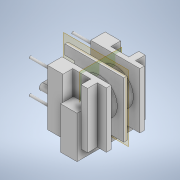
# Autodesk Inventor part: UU10.5Y
Saved by Autodesk Inventor 2020 (Build 240168000, 168)
## iProperties
Created: 2021-07-21
Part Number: UU10.5Y
Material: Типовые
Document SubType Name: Modeling
Designer: VB
Density: 1 g/cm^3
Appearance: По умолчанию
Author: VB
Autodesk Inventor part; units mm, degrees
ref_plane "YZ Plane" through (0, 0, 0) normal (1, 0, 0) x (0, 1, 0)
ref_plane "XZ Plane" through (0, 0, 0) normal (0, 1, 0) x (-1, 0, 0)
ref_plane "XY Plane" through (0, 0, 0) normal (0, 0, 1) x (1, 0, 0)
sketch "Эскиз1" plane through (0, 0, 0) normal (0, 1, 0) x (-1, 0, 0)
  line L0 (9, 8.8) -> (9, -8.8) construction
  line L1 (-9, -8.8) -> (-9, 8.8) construction
  line L2 (-9, 8.8) -> (9, -8.8) construction
  line L3 (9, 8.8) -> (-9, -8.8) construction
  line L4 (9, 0) -> (9, 0.5)
  line L5 (9, 0.5) -> (-9, 0.5)
  line L6 (9, 0) -> (9, -0.4719)
  line L7 (9, -0.4719) -> (-9, -0.4719)
  line L8 (-9, 0.5) -> (-9, -0.4719)
  line L9 (9, 0) -> (9, 4.3404) construction
  line L10 (9, 0) -> (9, -4.4046) construction
  line L11 (9, 4.3404) -> (-9, 4.3404)
  line L12 (-9, 4.3404) -> (-9, 8.8)
  line L13 (-9, 8.8) -> (9, 8.8)
  line L14 (9, 8.8) -> (9, 4.3404)
  line L15 (9, -4.4046) -> (-9, -4.4046)
  line L16 (-9, -4.4046) -> (-9, -8.8)
  line L17 (-9, -8.8) -> (9, -8.8)
  line L18 (9, -8.8) -> (9, -4.4046)
  point P0 (0, 0)
  dimension "d0" = 18
  dimension "d1" = 17.6
  dimension "d2" = 0.5
  constraints: 38 end point, 6 point on line, 5 parallel, 4 perpendicular, 3 midpoint, 2 horizontal, 1 collinear
  measures "d0" distance of L0.end L1.start
  measures "d1" distance of L0.start L0.end
  measures "d2" distance of L4.start L4.end
extrude "Выдавливание1" add sketch "Эскиз1" along normal blind 17
sketch "Эскиз6" plane through (9, 0, 4.3404) normal (0, 0, -1) x (-1, 0, 0)
  line L0 (9, 0) -> (9, 17) construction
  line L1 (18, 17) -> (0, 17) projected
  line L2 (9, 8.5) -> (7.5, 8.5) construction
  circle A0 centre (7.5, 8.5) radius 5.5
  dimension "d16" = 1.5
  dimension "d53" = 11
  constraints: 4 end point, 2 midpoint, 1 centre point, 1 coincident, 1 horizontal
  measures "d16" distance of L2.start L2.end
  measures "d53" diameter of A0
extrude "Выдавливание3" add sketch "Эскиз6" along normal up to surface (8.745 mm away)
sketch "Эскиз10" plane through (-9, 0, 4.3404) normal (-1, 0, 0) x (0, 0, 1)
  line L0 (4.4596, 6.45) -> (4.4596, 11.95) projected
  line L1 (4.4596, 9.2) -> (-13.9375, 9.2) construction
  line L2 (-14.0763, 11.7) -> (-14.0763, 6.7) projected
  line L3 (1, 9.2) -> (2.9596, 9.2) construction
  line L4 (1, 8.2) -> (2.9596, 8.2)
  line L5 (2.9596, 10.2) -> (1, 10.2)
  arc A0 (1, 10.2) -> (1, 8.2) centre (1, 9.2) ccw
  arc A1 (2.9596, 8.2) -> (2.9596, 10.2) centre (2.9596, 9.2) ccw
  line L6 (0, 0) -> (0, 17) projected
  line L7 (4.4596, 0) -> (4.4596, 17) projected
  line L8 (-9.745, 9.2) -> (-11.6404, 9.2) construction
  line L9 (-9.745, 10.2) -> (-11.6404, 10.2)
  line L10 (-11.6404, 8.2) -> (-9.745, 8.2)
  arc A2 (-9.745, 8.2) -> (-9.745, 10.2) centre (-9.745, 9.2) ccw
  arc A3 (-11.6404, 10.2) -> (-11.6404, 8.2) centre (-11.6404, 9.2) ccw
  line L11 (-8.745, 0) -> (-8.745, 17) projected
  line L12 (-13.1404, 0) -> (-13.1404, 17) projected
  line L13 (-4.8123, 0) -> (-4.8123, 17) projected
  line L14 (-3.8404, 0) -> (-3.8404, 3) projected
  line L15 (-4.8123, 0) -> (-3.8404, 0)
  line L16 (-3.8404, 0) -> (-3.8404, 3)
  line L17 (-3.8404, 3) -> (-4.8123, 3)
  line L18 (-4.8123, 3) -> (-4.8123, 0)
  line L19 (-4.8123, 0) -> (-4.8123, 17) projected
  line L20 (-3.8404, 17) -> (-4.8123, 17)
  line L21 (-4.8123, 17) -> (-4.8123, 14)
  line L22 (-4.8123, 14) -> (-3.8404, 14)
  line L23 (-3.8404, 14) -> (-3.8404, 17)
  line L24 (8.1135, -3.7823) -> (-17.89, -3.7823)
  line L25 (-17.89, -3.7823) -> (-17.89, 22.1054)
  line L26 (-17.89, 22.1054) -> (8.1135, 22.1054)
  line L27 (8.1135, 22.1054) -> (8.1135, -3.7823)
  point P0 (-4.3404, 0)
  point P1 (1.9798, 9.2)
  point P2 (-10.6927, 9.2)
  point P3 (-4.8123, 16.85)
  point P4 (-4.8123, 3)
  dimension "d44" = 2
  dimension "d45" = 1
  dimension "d46" = 1.5
  dimension "d47" = 1
  dimension "d48" = 1.5
  dimension "d49" = 3
  dimension "d50" = 3
  constraints: 42 end point, 8 parallel, 8 point on circle, 8 tangent, 5 point on line, 4 centre point, 4 perpendicular, 3 horizontal, 3 midpoint
  measures "d44" diameter of A1
  measures "d45" distance from line of L6 L3.start
  measures "d46" distance from line of L7 L3.end
  measures "d47" distance from line of L11 L8.start
  measures "d48" distance from line of L12 L8.end
  measures "d49" distance of L14.end L15.end
  measures "d50" distance of L21.end L20.end
extrude "Выдавливание6" cut sketch "Эскиз10" against normal blind 3
sketch "Эскиз11" plane through (-6, 0, 4.3404) normal (-1, 0, 0) x (0, 0, 1)
  line L0 (-4.3263, -2.8057) -> (-4.3263, 20.2349) construction
  line L1 (5.7896, 9.2) -> (-19.3839, 9.2) construction
  line L2 (2.1737, 14.2) -> (-10.8263, 14.2) construction
  line L3 (-10.8263, 14.2) -> (-10.8263, 4.2) construction
  line L4 (-10.8263, 4.2) -> (2.1737, 4.2) construction
  line L5 (2.1737, 4.2) -> (2.1737, 14.2) construction
  line L6 (2.1737, 14.2) -> (-10.8263, 4.2) construction
  line L7 (-10.8263, 14.2) -> (2.1737, 4.2) construction
  circle A0 centre (2.1737, 4.2) radius 0.35
  circle A1 centre (-10.8263, 4.2) radius 0.35
  circle A2 centre (-10.8263, 14.2) radius 0.35
  circle A3 centre (2.1737, 14.2) radius 0.35
  point P0 (-4.3404, 0)
  point P1 (-4.3263, 9.2)
  dimension "d54" = 13
  dimension "d55" = 10
  dimension "d56" = 0.7
  dimension "d57" = 0.7
  dimension "d58" = 0.7
  dimension "d59" = 0.7
  constraints: 16 end point, 4 centre point, 4 coincident, 2 horizontal, 2 midpoint, 2 parallel, 2 point on line, 1 perpendicular, 1 vertical
  measures "d54" distance of L4.end L3.end
  measures "d55" distance of L3.end L2.end
  measures "d56" diameter of A0
  measures "d57" diameter of A1
  measures "d58" diameter of A2
  measures "d59" diameter of A3
extrude "Выдавливание7" add sketch "Эскиз11" along normal blind 7.5
sketch "Эскиз12" plane through (9, 0, -8.8) normal (0, 0, -1) x (-1, 0, 0)
  line L0 (10.25, -3.9451) -> (4.75, -3.9451)
  line L1 (4.75, -3.9451) -> (4.75, 20.9451)
  line L2 (4.75, 20.9451) -> (10.25, 20.9451)
  line L3 (10.25, 20.9451) -> (10.25, -3.9451)
  circle A0 centre (7.5, 8.5) radius 5.5 projected
  line L4 (10.25, -3.9451) -> (4.75, 20.9451) construction
  line L5 (4.75, -3.9451) -> (10.25, 20.9451) construction
  line L6 (-8.7801, -3.9451) -> (2.75, -3.9451)
  line L7 (2.75, -3.9451) -> (2.75, 20.9451)
  line L8 (2.75, 20.9451) -> (-8.7801, 20.9451)
  line L9 (-8.7801, 20.9451) -> (-8.7801, -3.9451)
  line L10 (-8.7801, -3.9451) -> (2.75, 20.9451) construction
  line L11 (2.75, -3.9451) -> (-8.7801, 20.9451) construction
  point P0 (9, 0)
  point P1 (-3.0151, 8.5)
  dimension "d62" = 5.5
  dimension "d63" = 2
  constraints: 24 end point, 4 midpoint, 4 parallel, 2 horizontal, 2 perpendicular
  measures "d62" distance of L1.end L2.end
  measures "d63" distance between parallel lines of L1 L7
ref_plane "РабПлоскость3" through (9, 0, 0.014) normal (0, 0, 1) x (0, 1, 0)
extrude "Выдавливание8" cut sketch "Эскиз12" against normal blind 3 contours L0 L1 A0 L3 | A0 L1 L3 | A0 L1 L2 L3 | L7 L6 L9 L8 A0 | A0 L7
mirror "Зеркальное отражение1" about plane through (9, 0, 0.014) normal (0, 0, 1) of "Выдавливание8"
ref_plane "РабПлоскость4" through (1.5, 17, -5.8) normal (-1, 0, 0) x (0, -1, 0)
sketch "Эскиз14" plane through (6.25, 0, -8.8) normal (0, 0, -1) x (-1, 0, 0)
  line L0 (7.5, 0) -> (2, 0) projected
  line L1 (2, 0) -> (7.5, 0)
  line L2 (7.5, 0) -> (7.5, 3)
  line L3 (7.5, 3) -> (2, 3)
  line L4 (2, 3) -> (2, 0)
  point P0 (6.25, 0)
  dimension "d76" = 3
  constraints: 8 end point, 2 parallel, 1 horizontal, 1 perpendicular
  measures "d76" distance of L2.end L1.end
extrude "Выдавливание9" cut sketch "Эскиз14" against normal blind 23
sketch "Эскиз13" plane through (1.5, 17, -5.8) normal (-1, 0, 0) x (0, -1, 0)
  line L0 (20, -3.936) -> (7.2, -3.936)
  line L1 (7.2, -3.936) -> (7.2, 15.564)
  line L2 (7.2, 15.564) -> (20, 15.564)
  line L3 (20, 15.564) -> (20, -3.936)
  line L4 (20, -3.936) -> (7.2, 15.564) construction
  line L5 (7.2, -3.936) -> (20, 15.564) construction
  line L6 (16, -0.2) -> (11.2, -0.2)
  line L7 (11.2, -0.2) -> (11.2, 11.8281)
  line L8 (11.2, 11.8281) -> (16, 11.8281)
  line L9 (16, 11.8281) -> (16, -0.2)
  line L10 (16, -0.2) -> (11.2, 11.8281) construction
  line L11 (11.2, -0.2) -> (16, 11.8281) construction
  line L12 (0, 11.6281) -> (17, 11.6281) projected
  line L13 (17, 0) -> (0, 0) projected
  line L14 (11.2, 5.814) -> (7.2, 5.814) construction
  line L15 (9.2, 5.814) -> (9.2, 20.2386) construction
  line L16 (9.2, 13.0263) -> (9.2, 30.8178) construction
  point P0 (17, 5.8)
  point P1 (13.6, 5.814)
  point P2 (0, -3)
  point P3 (0, 14.6)
  point P4 (0, 10.1404)
  point P5 (11.2, 0)
  point P6 (7.2, 0)
  point P7 (7.2, 11.6281)
  point P8 (11.2, 11.6281)
  dimension "d66" = 0.2
  dimension "d67" = 0.2
  dimension "d68" = 4
  dimension "d69" = 19.5
  dimension "d70" = 20
  dimension "d73" = 9.2
  dimension "d75" = 0
  constraints: 30 end point, 7 midpoint, 4 parallel, 2 horizontal, 2 perpendicular, 2 vertical
  measures "d66" distance between parallel lines of L12 L8
  measures "d67" distance between parallel lines of L13 L6
  measures "d68" distance between parallel lines of L9 L3
  measures "d69" distance between parallel lines of L0 L2
  measures "d70" distance from line of point (0, -3) L3
  measures "d73" distance from line of point (0, 10.14) L16
  measures "d75" distance between parallel lines of L16 L15
extrude "Выдавливание10" add sketch "Эскиз13" along normal mid plane 5 contours L0 L1 L13 L7 L6 L9 L8 L12 L2 L3
sketch "Эскиз15" plane through (-6, 0, 4.3404) normal (-1, 0, 0) x (0, 0, 1)
  line L0 (-13.1404, 0) -> (-10.1404, 0) construction
  line L1 (-11.1404, 0) -> (-13.1404, 2)
  line L2 (-11.1404, 0) -> (-8.3119, 0) construction
  line L3 (-13.1404, 2) -> (-13.1404, 0)
  line L4 (-13.1404, 0) -> (-11.1404, 0)
  line L5 (-13.1404, 0) -> (-13.1404, 17) projected
  line L6 (-13.1404, 0) -> (-11.1404, 0)
  point P0 (-4.3404, 0)
  dimension "d81" = 135
  dimension "d82" = 2
  constraints: 10 end point, 1 collinear, 1 equal length, 1 horizontal, 1 perpendicular, 1 point on line, 1 vertical
  measures "d81" angle of L2 L1
  measures "d82" distance from line of L0 L1.end
extrude "Выдавливание11" cut sketch "Эскиз15" against normal up to surface (4.75 mm away)
